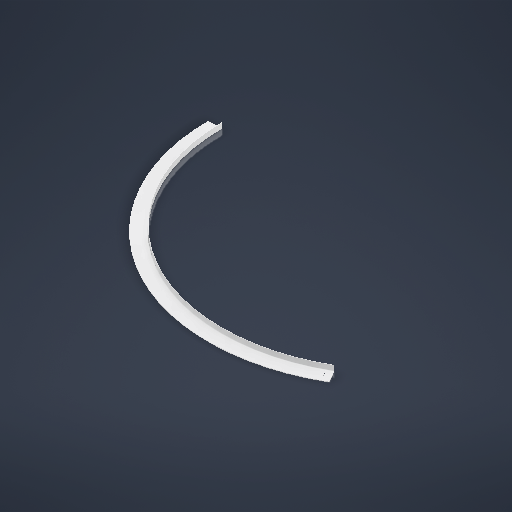
# Autodesk Inventor part: Support Ring Section, L Section
Saved by Autodesk Inventor 2026 (Build 300175000, 175)
## iProperties
Created: 2025-11-03
Part Number: Support Ring Section, L Section
Material: Aluminum 6061
Document SubType Name: Modeling
Designer: Brandon Portillo
Density: 2.7 g/cm^3
Appearance: Aluminum - Flat
Author: Brandon Portillo
Autodesk Inventor part; units mm, degrees
ref_plane "YZ Plane" through (0, 0, 0) normal (1, 0, 0) x (0, 1, 0)
ref_plane "XZ Plane" through (0, 0, 0) normal (0, 1, 0) x (-1, 0, 0)
ref_plane "XY Plane" through (0, 0, 0) normal (0, 0, 1) x (1, 0, 0)
sketch "Sketch1" plane through (0, 0, 0) normal (0, 0, 1) x (1, 0, 0)
  line L0 (-1950, 0) -> (-2090, 0)
  line L1 (0, 0) -> (0, 620.2794)
  line L2 (-2090, 0) -> (-1940, 0)
  line L3 (-1940, 0) -> (-1940, 6)
  line L4 (-1956, 6) -> (-2090, 6)
  line L5 (-2090, 6) -> (-2090, 0)
  line L6 (-1940, 0) -> (-2023.1832, 0)
  line L7 (-1946, 16) -> (-1946, 63.5827)
  line L8 (-1946, 63.5827) -> (-1940, 63.5827)
  line L9 (-1940, 63.5827) -> (-1940, 10)
  arc A0 (-1956, 6) -> (-1946, 16) centre (-1956, 16) ccw
  arc A1 (-1950, 0) -> (-1940, 10) centre (-1950, 10) ccw
  dimension "d0" = 2090
  dimension "d1" = 150
  dimension "d2" = 6
  dimension "d3" = 6
  dimension "d4" = 100
  dimension "d5" = 10
  dimension "d6" = 10
  constraints: 20 end point, 4 parallel, 4 point on circle, 4 tangent, 3 horizontal, 2 centre point, 2 perpendicular, 2 point on line, 1 vertical
  measures "d0" distance of L1.start L0.end
  measures "d1" distance of L4.end L3.end
  measures "d2" distance of L3.end L2.end
  measures "d3" distance of L7.end L8.end
  measures "d4" distance of L6.end L7.end
  measures "d5" radius of A0
  measures "d6" radius of A1
revolve "Revolution1" add sketch "Sketch1" angle 120 about axis through (0, 0, 0) along (0, 1, 0)
sketch "Sketch2" plane through (-2090, 6, 0) normal (0, 1, 0) x (1, 0, 0)
  line L0 (3068, -1693.9457) -> (3135, -1809.9931) projected
  arc A0 (3076.0233, -1842.7854) -> (3135, -1809.9931) centre (2090, 0) ccw
  line L1 (2090, 0) -> (3076.0233, -1842.7854) construction
  line L2 (2090, 0) -> (3135, -1809.9931) construction
  arc A1 (0, 0) -> (3135, -1809.9931) centre (2090, 0) ccw projected
  line L3 (3076.0233, -1842.7854) -> (3013.2859, -1725.5349)
  line L4 (3044.6546, -1784.1601) -> (3028.1423, -1753.3001)
  line L5 (3044.6546, -1784.1601) -> (3061.167, -1815.0202)
  line L6 (2090, 0) -> (1045, -1809.9931)
  line L7 (2090, 0) -> (4180, 0) construction
  line L8 (67.5447, -65.3249) -> (102.5264, -64.195)
  line L9 (67.5447, -65.3249) -> (32.5629, -66.4548)
  point P0 (1.0894, -67.4714)
  point P1 (1.0894, -67.4714)
  dimension "d8" = 1.85
  dimension "d9" = 35
  dimension "d10" = 35
  dimension "d11" = 120
  constraints: 18 end point, 7 symmetric about line, 5 coincident, 4 point on circle, 4 point on line, 1 centre point, 1 equal length, 1 horizontal, 1 midpoint
  measures "d8" angle of L1 L2
  measures "d9" distance of L4.start L4.end
  measures "d10" distance of L4.start L5.end
  measures "d11" angle of L6 L7
hole "Hole1" at (954.6546, 6, 1784.1601) at (938.1423, 6, 1753.3001) at (971.167, 6, 1815.0202) direction (0, -1, 0) diameter 10.2 end through all
thread "Thread1" size "M10x1.5" class "6H" standard "ANSI Metric M Profile" full length
thread "Thread2" size "M10x1.5" class "6H" standard "ANSI Metric M Profile" full length
thread "Thread3" size "M11x1.5" class "6H" standard "ANSI Metric M Profile" full length
hole "Hole2" at (-2022.4553, 6, 65.3249) at (-2057.4371, 6, 66.4548) at (-1987.4736, 6, 64.195) direction (0, -1, 0) diameter 10.2 end through all
thread "Thread4" size "M10x1.5" class "6H" standard "ANSI Metric M Profile" full length
thread "Thread5" size "M10x1.5" class "6H" standard "ANSI Metric M Profile" full length
thread "Thread6" size "M10x1.5" class "6H" standard "ANSI Metric M Profile" full length
body "Solid1"
